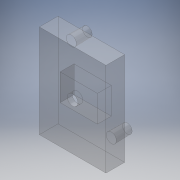
# Autodesk Inventor part: Base-Cover
Saved by Autodesk Inventor 2019 (Build 230136000, 136)
## iProperties
Created: 2021-01-07
Part Number: Base-Cover
Material: Polycarbonate, Clear
Document SubType Name: Modeling
Designer: Sam
Density: 1.2 g/cm^3
Appearance: Polycarbonate - Clear
Author: Sam
Autodesk Inventor part; units mm, degrees
ref_plane "YZ Plane" through (0, 0, 0) normal (1, 0, 0) x (0, 1, 0)
ref_plane "XZ Plane" through (0, 0, 0) normal (0, 1, 0) x (-1, 0, 0)
ref_plane "XY Plane" through (0, 0, 0) normal (0, 0, 1) x (1, 0, 0)
sketch "Sketch1" plane through (0, 0, 0) normal (0, 0, 1) x (1, 0, 0)
  line L0 (12.5, 17.5) -> (-12.5, 17.5) projected
  line L1 (-12.5, 17.5) -> (-12.5, -17.5) projected
  line L2 (12.5, -17.5) -> (12.5, 17.5) projected
  line L3 (-12.5, -17.5) -> (12.5, -17.5) projected
  circle A0 centre (0, 0) radius 2
  dimension "d0" = 4
  constraints: 1 centre point, 1 coincident
  measures "d0" diameter of A0
extrude "Extrusion1" add sketch "Sketch1" along normal blind 7
sketch "Sketch2" plane through (0, 0, 0) normal (0, 0, -1) x (-1, 0, 0)
  circle A0 centre (7.5, 12) radius 2.1 projected
  circle A1 centre (-7.5, -12) radius 2.1 projected
  line L0 (6.5, 5) -> (-7.5, 5)
  line L1 (-7.5, 5) -> (-7.5, -5)
  line L2 (-7.5, -5) -> (6.5, -5)
  line L3 (6.5, -5) -> (6.5, 5)
  line L4 (-6.5, 4.5) -> (5.5, 4.5) construction
  line L5 (5.5, 4.5) -> (5.5, -4.5) construction
  line L6 (5.5, -4.5) -> (-6.5, -4.5) construction
  line L7 (-6.5, -4.5) -> (-6.5, 4.5) construction
  circle A2 centre (7.5, 12) radius 1.9
  circle A3 centre (-7.5, -12) radius 1.9
  point P0 (0, 0)
  dimension "d3" = 1
  dimension "d4" = 0.5
  dimension "d5" = 0.5
  dimension "d6" = 1
  dimension "d9" = 3.8
  constraints: 8 end point, 2 centre point, 2 coincident, 2 parallel, 1 equal radius, 1 horizontal, 1 perpendicular
  measures "d3" distance between parallel lines of L5 L3
  measures "d4" distance between parallel lines of L6 L2
  measures "d5" distance between parallel lines of L4 L0
  measures "d6" distance between parallel lines of L7 L1
  measures "d9" diameter of A2
extrude "Extrusion3" add sketch "Sketch2" along normal blind 6 draft -1 contours A2 | A3
sketch "Sketch3" plane through (0, 0, 0) normal (0, 0, -1) x (-1, 0, 0)
  line L0 (5.5, 4.5) -> (5.5, -4.5) construction
  line L1 (-6.5, 4.5) -> (5.5, 4.5) construction
  line L2 (-6.5, -4.5) -> (-6.5, 4.5) construction
  line L3 (5.5, -4.5) -> (-6.5, -4.5) construction
  line L4 (6.5, 5) -> (-7.5, 5)
  line L5 (-7.5, 5) -> (-7.5, -5)
  line L6 (-7.5, -5) -> (6.5, -5)
  line L7 (6.5, -5) -> (6.5, 5)
  point P0 (0, 0)
  dimension "d12" = 1
  dimension "d13" = 0.5
  dimension "d14" = 0.5
  dimension "d15" = 1
  constraints: 8 end point, 2 parallel, 1 horizontal, 1 perpendicular
  measures "d12" distance between parallel lines of L0 L7
  measures "d13" distance between parallel lines of L3 L6
  measures "d14" distance between parallel lines of L4 L1
  measures "d15" distance between parallel lines of L5 L2
extrude "Extrusion4" cut sketch "Sketch3" against normal blind 5.2
sketch "Sketch4" plane through (0, 0, 5.2) normal (0, 0, -1) x (-1, 0, 0)
  circle A0 centre (4, 0) radius 0.6105 projected
  circle A1 centre (-5, 0) radius 0.6105 projected
  circle A2 centre (4, 0) radius 0.5
  circle A3 centre (-5, 0) radius 0.5
  point P0 (0, 0)
  dimension "d18" = 1
  constraints: 4 coincident, 2 centre point, 1 equal radius
  measures "d18" diameter of A2
extrude "Extrusion5" add sketch "Sketch4" along normal blind 2 contours A2 | A3
fillet "Fillet1" radius 0.2 2 edges at (5.5, 0, 5.2) (-3.5, 0, 5.2)
fillet "Fillet2" radius 0.4 2 edges at (5.5, 0, 3.2) (-3.5, 0, 3.2)
fillet "Fillet3" radius 0.5 2 edges at (9.4, -12, 0) (-5.6, 12, 0)
body "Solid1"
